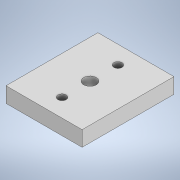
# Autodesk Inventor part: Shoulderbottom
Saved by Autodesk Inventor 2022 (Build 260153000, 153)
## iProperties
Created: 2022-03-24
Part Number: Shoulderbottom
Material: Genérico
Document SubType Name: Modeling
Designer: JK
Density: 1 g/cm^3
Appearance: Valor por defecto
Author: JK
Autodesk Inventor part; units mm, degrees
ref_plane "YZ Plane" through (0, 0, 0) normal (1, 0, 0) x (0, 1, 0)
ref_plane "XZ Plane" through (0, 0, 0) normal (0, 1, 0) x (-1, 0, 0)
ref_plane "XY Plane" through (0, 0, 0) normal (0, 0, 1) x (1, 0, 0)
sketch "Boceto1" plane through (0, 0, 0) normal (0, 1, 0) x (-1, 0, 0)
  line L0 (-24.85, 30) -> (24.85, 30)
  line L1 (24.85, 30) -> (24.85, -30)
  line L2 (24.85, -30) -> (-24.85, -30)
  line L3 (-24.85, -30) -> (-24.85, 30)
  line L4 (-24.85, 30) -> (24.85, -30) construction
  line L5 (24.85, 30) -> (-24.85, -30) construction
  circle A0 centre (0, 0) radius 4.15
  circle A1 centre (0, 18.25) radius 2.7
  circle A2 centre (0, -18.25) radius 2.7
  dimension "d0" = 49.7
  dimension "d1" = 8.3
  dimension "d2" = 60
  dimension "d3" = 5.4
  dimension "d4" = 5.4
  dimension "d5" = 18.25
  dimension "d6" = 36.5
  constraints: 12 end point, 3 centre point, 2 midpoint, 2 parallel, 1 coincident, 1 horizontal, 1 perpendicular
  measures "d0" distance of L0.start L0.end
  measures "d1" diameter of A0
  measures "d2" distance of L0.end L1.end
  measures "d3" diameter of A1
  measures "d4" diameter of A2
  measures "d5" distance of point (0, 0) A1.centre
  measures "d6" distance of A2.centre A1.centre
extrude "Extrusión1" add sketch "Boceto1" along normal blind 10
